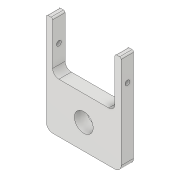
# Autodesk Inventor part: Needle Bearing Mount
Saved by Autodesk Inventor 2018.3 (Build 223284000, 284)
## iProperties
Created: 2018-12-21
Part Number: Needle Bearing Mount
Material: ABS Plastic
Document SubType Name: Modeling
Designer: aye06091
Mass: 56.6258 g
Surface Area: 149.687 cm^2
Volume: 53.4206 cm^3
Density: 1.06 g/cm^3
Appearance: Smooth - White
Author: aye06091
Autodesk Inventor part; units mm, degrees
note: some values were not read from the file. Chosen so that the rebuilt part matches the saved one: sketch regions of "Extrusion1".
ref_plane "YZ Plane" through (0, 0, 0) normal (1, 0, 0) x (0, 1, 0)
ref_plane "XZ Plane" through (0, 0, 0) normal (0, 1, 0) x (-1, 0, 0)
ref_plane "XY Plane" through (0, 0, 0) normal (0, 0, 1) x (1, 0, 0)
sketch "Sketch1" plane through (0, 0, 0) normal (0, 0, 1) x (1, 0, 0)
  line L0 (0, 0) -> (50.8, 0)
  line L1 (50.8, 0) -> (50.8, -50.8)
  line L2 (50.8, -50.8) -> (0, -50.8)
  line L3 (0, -50.8) -> (0, 0)
  circle A0 centre (25.4, -25.4) radius 9.5885
  line L4 (0, -50.8) -> (-12.7, -50.8)
  line L5 (-12.7, -50.8) -> (-12.7, 50.8)
  line L6 (-12.7, 50.8) -> (-6.35, 50.8)
  line L7 (0, 0) -> (0, -50.8)
  line L8 (50.8, -50.8) -> (63.5, -50.8)
  line L9 (63.5, -50.8) -> (63.5, 50.8)
  line L10 (63.5, 50.8) -> (57.15, 50.8)
  line L11 (50.8, 0) -> (50.8, -50.8)
  line L12 (-6.35, 50.8) -> (-6.35, 0)
  line L13 (-6.35, 0) -> (0, 0)
  line L14 (57.15, 50.8) -> (57.15, 0)
  line L15 (57.15, 0) -> (50.8, 0)
  dimension "d0" = 19.177
  dimension "d1" = 50.8
  dimension "d2" = 50.8
  dimension "d37" = 25.4
  dimension "d44" = 101.6
  dimension "d45" = 101.6
  constraints: 32 end point, 6 parallel, 3 horizontal, 3 perpendicular, 1 centre point, 1 point on line
  measures "d0" diameter of A0
  measures "d1" distance of L0.end L1.end
  measures "d2" distance of L1.end L2.end
  measures "d37" distance from line of A0.centre L2
  measures "d44" distance of L4.end L5.end
  measures "d45" distance of L8.end L9.end
extrude "Extrusion1" add sketch "Sketch1" against normal blind 12.7
sketch "Sketch9" plane through (63.5, -50.8, 0) normal (1, 0, 0) x (0, 0, -1)
  line L0 (0, 101.6) -> (0, 0) projected
  line L1 (0, 101.6) -> (12.7, 101.6) projected
  circle A0 centre (6.35, 76.2) radius 2.4447
  point P0 (0, 50.8)
  dimension "d48" = 4.8895
  dimension "d49" = 6.35
  dimension "d50" = 25.4
  constraints: 1 centre point
  measures "d48" diameter of A0
  measures "d49" distance from line of L0 A0.centre
  measures "d50" distance from line of L1 A0.centre
extrude "Extrusion9" cut sketch "Sketch9" against normal through all
fillet "Fillet13" radius 1.5875 4 edges at (-12.7, 50.8, -6.35) (-6.35, 50.8, -6.35) (57.15, 50.8, -6.35) (63.5, 50.8, -6.35)
fillet "Fillet14" radius 6.35 4 edges at (63.5, -50.8, -6.35) (-12.7, -50.8, -6.35) (-6.35, 0, -6.35) (57.15, 0, -6.35)
body "Solid1"
